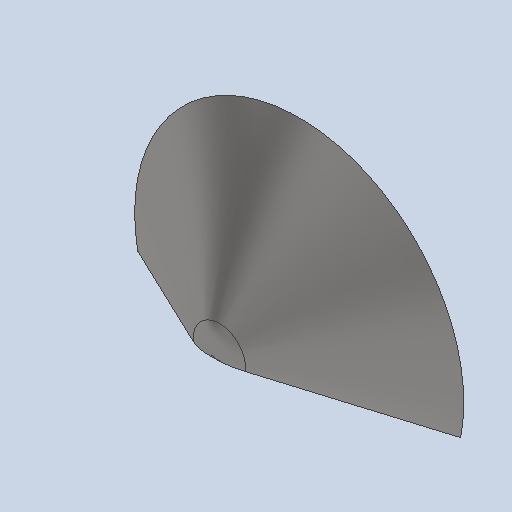
# Autodesk Inventor part: nose
Saved by Autodesk Inventor 2024 (Build 280153000, 153)
## iProperties
Created: 2023-06-07
Part Number: nose
Material: Steel, Mild
Document SubType Name: Modeling
Designer: tamiz
Density: 7.85 g/cm^3
Appearance: Semi-Polished
Author: tamiz
Autodesk Inventor part; units mm, degrees
ref_plane "YZ Plane" through (0, 0, 0) normal (1, 0, 0) x (0, 1, 0)
ref_plane "Work Plane8" through (0, -1837.3344, 10759.44) normal (0, 0, 1) x (-0.6391035, -0.7691208, 0)
sketch "Sketch14" plane through (0, -1837.3344, 10759.44) normal (0, 0, 1) x (-0.6391035, -0.7691208, 0)
  arc A0 (51.9231, 278.7941) -> (283.588, 0) centre (141.794, 117.8242) ccw projected
  arc A1 (128.7949, 130.8233) -> (154.7931, 104.8251) centre (141.794, 117.8242) ccw
  line L0 (141.794, 117.8242) -> (128.7949, 130.8233)
  line L1 (128.7949, 130.8233) -> (154.7931, 104.8251)
  point P0 (-1413.132, -1174.2468)
  constraints: 4 end point, 2 point on circle, 1 centre point, 1 coincident
extrude "Extrusion9" add sketch "Sketch14" against normal blind 106.68 draft 60
ref_plane "Work Plane9" through (0, -2021.693, 10759.44) normal (0, -0.9381218, 0.3463054) x (-0.8718495, -0.1696114, -0.4594676)
sketch "Sketch15" plane through (0, -2021.693, 10759.44) normal (0, -0.9381218, 0.3463054) x (-0.8718495, -0.1696114, -0.4594676)
  line L0 (-172.5198, -77.543) -> (270.8607, -77.543)
  line L1 (270.8607, -77.543) -> (270.8607, 243.8061)
  line L2 (270.8607, 243.8061) -> (-172.5198, 243.8061)
  line L3 (-172.5198, 243.8061) -> (-172.5198, -77.543)
  point P0 (4600.712, 8189.7549)
  constraints: 8 end point, 2 parallel, 1 horizontal, 1 perpendicular
extrude "Extrusion10" cut sketch "Sketch15" along normal blind 304.8
fillet "Fillet5" radius 60.96 1 edges at (-0.8449, -2003.3289, 10759.44)
body "Solid1"
